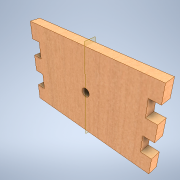
# Autodesk Inventor part: Front
Saved by Autodesk Inventor 2021.2 (Build 252289000, 289)
## iProperties
Created: 2021-03-04
Part Number: Front
Material: Wood (Cherry)
Document SubType Name: Modeling
Designer: 443201246
Density: 0.63 g/cm^3
Appearance: Cherry - Natural Low Gloss
Author: 443201246
Autodesk Inventor part; units mm, degrees
ref_plane "YZ Plane" through (0, 0, 0) normal (1, 0, 0) x (0, 1, 0)
ref_plane "XZ Plane" through (0, 0, 0) normal (0, 1, 0) x (-1, 0, 0)
ref_plane "XY Plane" through (0, 0, 0) normal (0, 0, 1) x (1, 0, 0)
sketch "Sketch1" plane through (0, 0, 0) normal (0, 0, 1) x (1, 0, 0)
  line L0 (0, 0) -> (164, 0)
  line L1 (164, 0) -> (164, 100)
  line L2 (164, 100) -> (0, 100)
  line L3 (0, 100) -> (0, 0)
  dimension "d0" = 164
  dimension "d1" = 100
  constraints: 8 end point, 2 parallel, 1 horizontal, 1 perpendicular
  measures "d0" distance of L2.end L1.end
  measures "d1" distance of L1.end L0.end
extrude "Extrusion1" add sketch "Sketch1" along normal blind 12
sketch "Sketch2" plane through (0, 0, 12) normal (0, 0, 1) x (1, 0, 0)
  line L0 (0, 100) -> (0, 0) projected
  line L1 (164, 100) -> (0, 100) projected
  line L2 (0, 100) -> (0, 0) projected
  line L3 (0, 20) -> (12, 20)
  line L4 (12, 20) -> (12, 40)
  line L5 (12, 40) -> (0, 40)
  line L6 (0, 40) -> (0, 20)
  line L7 (0, 0) -> (164, 0) projected
  line L8 (0, 60) -> (12, 60)
  line L9 (12, 60) -> (12, 80)
  line L10 (12, 80) -> (0, 80)
  line L11 (0, 80) -> (0, 60)
  point P0 (0, 40)
  dimension "d7" = 12
  dimension "d8" = 20
  dimension "d9" = 20
  dimension "d10" = 12
  dimension "d11" = 20
  dimension "d12" = 20
  constraints: 16 end point, 4 parallel, 2 horizontal, 2 perpendicular, 2 point on line
  measures "d7" distance of L5.end L4.end
  measures "d8" distance of L4.end L3.end
  measures "d9" distance between parallel lines of L3 L7
  measures "d10" distance of L10.end L9.end
  measures "d11" distance of L9.end L8.end
  measures "d12" distance between parallel lines of L8 L5
extrude "Extrusion2" cut sketch "Sketch2" against normal through all
ref_plane "Work Plane1" through (82, 0, 0) normal (1, 0, 0) x (0, 0, -1)
mirror "Mirror1" about plane through (82, 0, 0) normal (1, 0, 0) of "Extrusion2"
sketch "Sketch6" plane through (0, 0, 12) normal (0, 0, 1) x (1, 0, 0)
  circle A0 centre (82, 50) radius 5
  line L0 (0, 60) -> (0, 40) projected
  line L1 (0, 0) -> (164, 0) projected
  dimension "d25" = 10
  dimension "d26" = 82
  dimension "d27" = 50
  constraints: 1 centre point
  measures "d25" diameter of A0
  measures "d26" distance from line of L0 A0.centre
  measures "d27" distance from line of L1 A0.centre
extrude "Extrusion5" cut sketch "Sketch6" against normal through all
body "Solid1"
